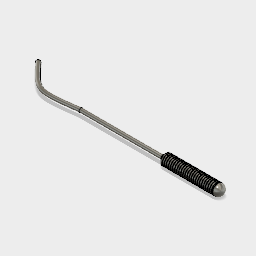
Prostate_Boundary_Detection_Internal v3 (Autodesk Fusion 360 design; units mm, degrees)
Autodesk Fusion 360 part; units mm, degrees
sketch "Sketch1" plane through (0, 0, 0) normal (0, 1, 0) x (1, 0, 0)
  line L0 (-13.444327, 0.5) -> (16.555673, 0.5)
  line L1 (16.555673, 0.5) -> (16.555673, 0.75)
  line L2 (16.555673, 0.75) -> (-13.444327, 0.75)
  line L3 (-13.444327, 0.75) -> (-13.444327, 0.5)
  dimension "d2" = 30
  dimension "d4" = 0.5
  dimension "d5" = 0.25
  measures "d4" distance of origin L0
revolve "Revolve1" add sketch "Sketch1" angle 360 about axis through (1.75, 0, 0) along (1, 0, 0) makes body 1
cylinder "CylinderPrimitive1" add diameter 4 height 20 placed x (0, 0, -1) y (0, 1, 0) z (1, 0, 0) at (16.555673, 0, 0) bodies 1
sphere "SpherePrimitive1" add diameter 4 placed x (0, 0, -1) y (0, 1, 0) z (1, 0, 0) at (36.555673, 0, 0) separate body makes body 2
chamfer "Chamfer1" distance 1 angle 45 1 edges at (16.555673, 0.723231, 1.864655) on bodies 1
sketch "Sketch5" plane through (0, 0, 0) normal (0, 0, 1) x (1, 0, 0)
  line L0 (18, 2) -> (18.2, 2)
  line L1 (18.2, 2) -> (18.2, 1.9)
  line L2 (18.2, 1.9) -> (18, 1.9)
  line L3 (18, 1.9) -> (18, 2)
  line L4 (18.95, 2) -> (18.95, 1.9)
  line L5 (18.75, 2) -> (18.95, 2)
  line L6 (18.75, 1.9) -> (18.75, 2)
  line L7 (18.95, 1.9) -> (18.75, 1.9)
  line L8 (19.7, 2) -> (19.7, 1.9)
  line L9 (19.5, 2) -> (19.7, 2)
  line L10 (19.5, 1.9) -> (19.5, 2)
  line L11 (19.7, 1.9) -> (19.5, 1.9)
  line L12 (20.45, 2) -> (20.45, 1.9)
  line L13 (20.25, 2) -> (20.45, 2)
  line L14 (20.25, 1.9) -> (20.25, 2)
  line L15 (20.45, 1.9) -> (20.25, 1.9)
  line L16 (21.2, 2) -> (21.2, 1.9)
  line L17 (21, 2) -> (21.2, 2)
  line L18 (21, 1.9) -> (21, 2)
  line L19 (21.2, 1.9) -> (21, 1.9)
  line L20 (21.95, 2) -> (21.95, 1.9)
  line L21 (21.75, 2) -> (21.95, 2)
  line L22 (21.75, 1.9) -> (21.75, 2)
  line L23 (21.95, 1.9) -> (21.75, 1.9)
  line L24 (22.7, 2) -> (22.7, 1.9)
  line L25 (22.5, 2) -> (22.7, 2)
  line L26 (22.5, 1.9) -> (22.5, 2)
  line L27 (22.7, 1.9) -> (22.5, 1.9)
  line L28 (23.45, 2) -> (23.45, 1.9)
  line L29 (23.25, 2) -> (23.45, 2)
  line L30 (23.25, 1.9) -> (23.25, 2)
  line L31 (23.45, 1.9) -> (23.25, 1.9)
  line L32 (24.2, 2) -> (24.2, 1.9)
  line L33 (24, 2) -> (24.2, 2)
  line L34 (24, 1.9) -> (24, 2)
  line L35 (24.2, 1.9) -> (24, 1.9)
  line L36 (24.95, 2) -> (24.95, 1.9)
  line L37 (24.75, 2) -> (24.95, 2)
  line L38 (24.75, 1.9) -> (24.75, 2)
  line L39 (24.95, 1.9) -> (24.75, 1.9)
  line L40 (25.7, 2) -> (25.7, 1.9)
  line L41 (25.5, 2) -> (25.7, 2)
  line L42 (25.5, 1.9) -> (25.5, 2)
  line L43 (25.7, 1.9) -> (25.5, 1.9)
  line L44 (26.45, 2) -> (26.45, 1.9)
  line L45 (26.25, 2) -> (26.45, 2)
  line L46 (26.25, 1.9) -> (26.25, 2)
  line L47 (26.45, 1.9) -> (26.25, 1.9)
  line L48 (27.2, 2) -> (27.2, 1.9)
  line L49 (27, 2) -> (27.2, 2)
  line L50 (27, 1.9) -> (27, 2)
  line L51 (27.2, 1.9) -> (27, 1.9)
  line L52 (27.95, 2) -> (27.95, 1.9)
  line L53 (27.75, 2) -> (27.95, 2)
  line L54 (27.75, 1.9) -> (27.75, 2)
  line L55 (27.95, 1.9) -> (27.75, 1.9)
  line L56 (28.7, 2) -> (28.7, 1.9)
  line L57 (28.5, 2) -> (28.7, 2)
  line L58 (28.5, 1.9) -> (28.5, 2)
  line L59 (28.7, 1.9) -> (28.5, 1.9)
  line L60 (29.45, 2) -> (29.45, 1.9)
  line L61 (29.25, 2) -> (29.45, 2)
  line L62 (29.25, 1.9) -> (29.25, 2)
  line L63 (29.45, 1.9) -> (29.25, 1.9)
  line L64 (30.2, 2) -> (30.2, 1.9)
  line L65 (30, 2) -> (30.2, 2)
  line L66 (30, 1.9) -> (30, 2)
  line L67 (30.2, 1.9) -> (30, 1.9)
  line L68 (30.95, 2) -> (30.95, 1.9)
  line L69 (30.75, 2) -> (30.95, 2)
  line L70 (30.75, 1.9) -> (30.75, 2)
  line L71 (30.95, 1.9) -> (30.75, 1.9)
  line L72 (31.7, 2) -> (31.7, 1.9)
  line L73 (31.5, 2) -> (31.7, 2)
  line L74 (31.5, 1.9) -> (31.5, 2)
  line L75 (31.7, 1.9) -> (31.5, 1.9)
  line L76 (32.45, 2) -> (32.45, 1.9)
  line L77 (32.25, 2) -> (32.45, 2)
  line L78 (32.25, 1.9) -> (32.25, 2)
  line L79 (32.45, 1.9) -> (32.25, 1.9)
  line L80 (33.2, 2) -> (33.2, 1.9)
  line L81 (33, 2) -> (33.2, 2)
  line L82 (33, 1.9) -> (33, 2)
  line L83 (33.2, 1.9) -> (33, 1.9)
  line L84 (33.95, 2) -> (33.95, 1.9)
  line L85 (33.75, 2) -> (33.95, 2)
  line L86 (33.75, 1.9) -> (33.75, 2)
  line L87 (33.95, 1.9) -> (33.75, 1.9)
  line L88 (34.7, 2) -> (34.7, 1.9)
  line L89 (34.5, 2) -> (34.7, 2)
  line L90 (34.5, 1.9) -> (34.5, 2)
  line L91 (34.7, 1.9) -> (34.5, 1.9)
  line L92 (35.45, 2) -> (35.45, 1.9)
  line L93 (35.25, 2) -> (35.45, 2)
  line L94 (35.25, 1.9) -> (35.25, 2)
  line L95 (35.45, 1.9) -> (35.25, 1.9)
  line L96 (36.2, 2) -> (36.2, 1.9)
  line L97 (36, 2) -> (36.2, 2)
  line L98 (36, 1.9) -> (36, 2)
  line L99 (36.2, 1.9) -> (36, 1.9)
  dimension "d12" = 18
  dimension "d13" = 0
revolve "Revolve2" cut sketch "Sketch5" angle 360 about axis through (1.75, 0, 0) along (1, 0, 0) bodies 1 2
sketch "Sketch6" plane through (0, 0, 0) normal (0, 1, 0) x (1, 0, 0)
  spline S0 degree 2 poles (-13.444327, 0) (-28, -2) (-36.425906, 7.441653) knots 0 0 0 2.59945978 2.59945978 2.59945978 weights 1 3 1
  line L0 (-13.444327, -0.75) -> (-13.444327, 0.75)
sketch "Sketch7" plane through (-13.444327, 0, 0) normal (-1, 0, 0) x (0, 0, 1)
  circle A0 centre (0, 0) radius 0.5
  circle A1 centre (0, 0) radius 0.75
  circle A2 centre (0, 0) radius 0.75
  circle A3 centre (0, 0) radius 0.5
sweep "Sweep1" add profiles "Sketch7" path "Sketch6" along S0 section 1 separate body makes body 3
